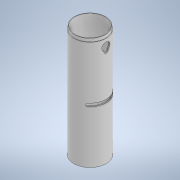
# Autodesk Inventor part: payloadchamber
Saved by Autodesk Inventor 2020.3 (Build 243373000, 373)
## iProperties
Created: 2021-01-23
Part Number: payloadchamber
Material: ABS Plastic
Document SubType Name: Modeling
Designer: 0x6f736f646f
Density: 1.06 g/cm^3
Appearance: Default
Author: 0x6f736f646f
Autodesk Inventor part; units mm, degrees
ref_plane "YZ Plane" through (0, 0, 0) normal (1, 0, 0) x (0, 1, 0)
ref_plane "XY Plane" through (0, 0, 0) normal (0, 0, 1) x (1, 0, 0)
sketch "Sketch1" plane through (0, 0, 0) normal (0, 1, 0) x (-1, 0, 0)
  circle A0 centre (0, 0) radius 25.9
  circle A1 centre (0, 0) radius 25
  circle A2 centre (0, 0) radius 26.8
  circle A3 centre (0, 0) radius 10
  dimension "d0" = 51.8
  dimension "d1" = 50
  dimension "d2" = 53.6
  dimension "d12" = 20
  constraints: 4 centre point, 4 coincident
  measures "d0" diameter of A0
  measures "d1" diameter of A1
  measures "d2" diameter of A2
  measures "d12" diameter of A3
extrude "Extrusion1" add sketch "Sketch1" along normal blind 95 and the other way blind 85 contours A0
extrude "Extrusion2" add sketch "Sketch1" along normal mid plane 180 contours A2
ref_plane "Work Plane1" through (0, 40, 0) normal (0, 1, 0) x (-1, 0, 0)
sketch "Sketch2" plane through (0, 40, 0) normal (0, 1, 0) x (-1, 0, 0)
  circle A0 centre (0, 0) radius 25.9
  circle A1 centre (0, 0) radius 25
  circle A2 centre (0, 0) radius 26.8
  circle A3 centre (0, 0) radius 10
  dimension "d14" = 51.8
  dimension "d15" = 50
  dimension "d16" = 53.6
  dimension "d17" = 20
  constraints: 4 centre point, 4 coincident
  measures "d14" diameter of A0
  measures "d15" diameter of A1
  measures "d16" diameter of A2
  measures "d17" diameter of A3
extrude "Extrusion3" add sketch "Sketch2" along normal blind 5 contours A1
sketch "Sketch3" plane through (0, 0, 0) normal (1, 0, 0) x (0, 1, 0)
  circle A0 centre (78.5, 0) radius 6.5
  circle A1 centre (72.5, 0) radius 3.5
  line L0 (90, -26.8) -> (90, 26.8) projected
  point P0 (0, 0)
  point P1 (73, 3.4641)
  point P2 (73, -3.4641)
  dimension "d20" = 13
  dimension "d21" = 7
  dimension "d22" = 11.5
  dimension "d23" = 16
  constraints: 2 centre point
  measures "d20" diameter of A0
  measures "d21" diameter of A1
  measures "d22" distance from line of A0.centre L0
extrude "Extrusion4" cut sketch "Sketch3" along normal blind 30
sketch "Sketch4" plane through (0, 0, 0) normal (1, 0, 0) x (0, 1, 0)
  line L0 (0, 20) -> (0, -20) construction
  line L1 (-2.5, 20) -> (-2.5, -20)
  line L2 (2.5, -20) -> (2.5, 20)
  arc A0 (2.5, 20) -> (-2.5, 20) centre (0, 20) ccw
  arc A1 (-2.5, -20) -> (2.5, -20) centre (0, -20) ccw
  point P0 (0, 0)
  point P1 (0, 0)
  dimension "d26" = 40
  dimension "d27" = 5
  constraints: 8 end point, 4 point on circle, 4 tangent, 2 centre point, 1 midpoint, 1 parallel, 1 vertical
  measures "d26" distance of L0.start L0.end
  measures "d27" diameter of A1
extrude "Extrusion5" cut sketch "Sketch4" along normal blind 30
body "Solid1"
